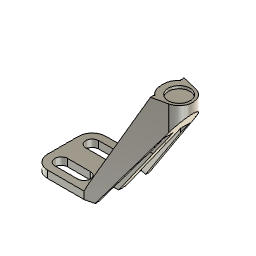
Melta holder for linear init with induction sensor (Autodesk Fusion 360 design; units mm, degrees)
Autodesk Fusion 360 part; units mm, degrees
sketch "Sketch1" plane through (0, 0, 0) normal (0, 0, 1) x (1, 0, 0)
  circle A0 centre (7.5, 6.1469) radius 3.5
  circle A1 centre (7.5, 23.1469) radius 3.5
  circle A2 centre (20, 23.1469) radius 3.5
  circle A3 centre (20, 6.1469) radius 3.5
  line L0 (0, 0) -> (0, 35)
  line L1 (7.5, 26.6469) -> (20, 26.6469)
  line L2 (7.5, 2.6469) -> (20, 2.6469)
  line L3 (7.5, 9.6469) -> (20, 9.6469)
  line L4 (7.5, 19.6469) -> (20, 19.6469)
  circle A4 centre (7.5, 23.1469) radius 7.5
  circle A5 centre (7.5, 6.1469) radius 7.5
  line L5 (0, 23.1469) -> (0, 6)
  circle A6 centre (20, 6.1469) radius 7.5
  circle A7 centre (20, 23.1469) radius 7.5
  line L6 (7.5, 30.6469) -> (20, 30.6469)
  line L7 (7.5, -1.3531) -> (20, -1.3531)
  line L8 (20, -1.3531) -> (27.5, -1.3531)
  line L9 (27.5, -1.3531) -> (27.5, 30.6469)
  line L10 (27.5, 30.6469) -> (20, 30.6469)
  circle A8 centre (63.75, 14.5734) radius 6
  line L11 (13.75, 19.6469) -> (13.75, 2.6469)
  circle A9 centre (63.75, 14.5734) radius 7.5
  line L12 (27.5, -1.3531) -> (65.4115, 7.2598)
  line L13 (27.5, 30.6469) -> (65.4384, 21.8809)
  line L14 (27.5, 14.6469) -> (56.2504, 14.6469)
  line L15 (27.5, 14.6469) -> (27.5, -1.3531)
  arc A10 (56.2504, 14.6469) -> (65.4115, 7.2598) centre (63.75, 14.5734) ccw
  arc A11 (65.4384, 21.8809) -> (56.2504, 14.6469) centre (63.75, 14.5734) ccw
  line L16 (27.5, 14.6469) -> (27.5, 30.6469)
  line L17 (29.5, 16.6469) -> (54.479, 16.6469)
  arc A12 (57.4411, 21.6761) -> (54.479, 16.6469) centre (63.75, 14.5734) ccw
  line L18 (29.5, 28.1321) -> (57.4411, 21.6761)
  line L19 (29.5, 16.6469) -> (29.5, 28.1321)
  line L20 (29.5, 1.1522) -> (57.415, 7.4941)
  arc A13 (54.4474, 12.6469) -> (57.415, 7.4941) centre (63.75, 14.5734) ccw
  line L21 (29.5, 12.6469) -> (54.4474, 12.6469)
  line L22 (29.5, 12.6469) -> (29.5, 1.1522)
  dimension "d1" = 7
  dimension "d2" = 7
  dimension "d3" = 17
  dimension "d4" = 7
  dimension "d5" = 7
  dimension "d8" = 7.5
  dimension "d9" = 7.5
  dimension "d10" = 20
  dimension "d11" = 20
  dimension "d12" = 15
  dimension "d13" = 15
  dimension "d14" = 15
  dimension "d15" = 15
  dimension "d16" = 7.5
  dimension "d17" = 12
  dimension "d19" = 50
  dimension "d20" = 15
  dimension "d21" = 2
  dimension "d22" = 2
  constraint coincident L0.start origin
  constraint vertical L0
  constraint coincident A1 L1.start
  constraint coincident A2 L1.end
  constraint tangent A2 L1
  constraint horizontal L1
  constraint coincident A0 L2.start
  constraint coincident A3 L2.end
  constraint tangent A3 L2
  constraint parallel L1 L2
  constraint coincident A0 L3.start
  constraint coincident A3 L3.end
  constraint tangent A3 L3
  constraint parallel L2 L3
  constraint coincident A1 L4.start
  constraint coincident A2 L4.end
  constraint tangent A2 L4
  constraint parallel L3 L4
  constraint concentric A1 A4
  constraint concentric A0 A5
  constraint coincident A4 L5.start
  constraint coincident L0 L5.end
  constraint tangent A4 L5
  constraint parallel L0 L5
  constraint concentric A3 A6
  constraint concentric A2 A7
  constraint coincident A4 L6.start
  constraint coincident A7 L6.end
  constraint tangent A7 L6
  constraint tangent A4 L6
  constraint coincident A5 L7.start
  constraint coincident A6 L7.end
  constraint tangent A6 L7
  constraint horizontal L7
  constraint parallel L7 L8
  constraint perpendicular L6 L9
  constraint tangent A7 L10
  constraint midpoint L4 L11.start
  constraint midpoint L2 L11.end
  constraint concentric A8 A9
  constraint coincident A9 L12.end
  constraint tangent A9 L12
  constraint coincident A9 L13.end
  constraint tangent A9 L13
  constraint midpoint L9 L14.start
  constraint coincident A9 L14.end
  constraint perpendicular L9 L14
  constraint coincident A8.centre A9.centre
  measures "d1" diameter of A0
  measures "d2" diameter of A1
  measures "d3" vertical distance of A0.centre A1.centre
  measures "d4" diameter of A2
  measures "d5" diameter of A3
  measures "d8" distance of A0.centre L0
  measures "d9" distance of A1.centre L0
  measures "d10" distance of A2.centre L0
  measures "d11" distance of A3.centre L0
  measures "d12" diameter of A4
  measures "d13" diameter of A5
  measures "d14" diameter of A6
  measures "d15" diameter of A7
  measures "d16" distance of L7.end L8.end
  measures "d17" diameter of A8
  measures "d19" distance of A8.centre L11
  measures "d20" diameter of A9
extrude "Extrude1" add sketch "Sketch1" along normal blind 4 contours A0 L2 L3 A5 A6 | L3 A6 L11 | L2 A5 A6 | L3 A5 L11 | A3 L2 L3 A5 A6 | A6 A7 L9 L11 L15 L16 | L0 A4 A5 L5 L11 | A5 A6 L7 | A6 L8 L9 L15 | L4 A4 L11 | A1 L1 L4 A4 A7 | A2 L1 L4 A4 A7 | L4 A7 L11 | A7 L9 L10 L16 | A4 A7 L6 | L1 A4 A7
extrude "Extrude2" add sketch "Sketch1" along normal blind 60 contours L9 A9 L12 L14 L15 A10 | L9 A9 L13 L14 A11 L16 | A9 A10 A11 | A8
chamfer "Chamfer1" distance 27 distance2 56 1 edges at (27.5, 14.6469, 60) measured on face at (61.7658, 13.9292, 60)
chamfer "Chamfer2" distance 57 distance2 2.7 2 edges at (54.5, 5.8064, 60) (54.5, 23.382, 60) measured on face at (28.1667, 15.3135, 5.3827) measured on face at (28.1667, 15.3135, 5.3827)
sketch "Sketch3" plane through (0, -1.3531, 0) normal (0, -1, 0) x (1, 0, 0)
  line L0 (7.5, 0) -> (27.5, 0)
  line L1 (27.5, 0) -> (27.5, 4)
  line L2 (27.5, 4) -> (7.5, 4)
  line L3 (7.5, 4) -> (7.5, 0)
  line L4 (32.4174, -0.0986) -> (71.6605, 55.2443)
  line L5 (71.6605, 55.2443) -> (71.6605, -0.0986)
  line L6 (71.6605, -0.0986) -> (32.4174, -0.0986)
  line L7 (71.6605, 55.2443) -> (78, 55.2443)
  line L8 (78, 55.2443) -> (78, 0)
  line L9 (78, 0) -> (71.6605, 0)
  line L10 (71.6605, 0) -> (71.6605, 55.2443)
  constraint perpendicular L2 L5
  constraint perpendicular L5 L6
  constraint horizontal L7
  constraint vertical L8
  constraint horizontal L9
  constraint vertical L10
extrude "Extrude4" cut sketch "Sketch3" against normal blind 40 contours L4 L5 L6 L10 | L5 L7 L8 L9 L10
sketch "Sketch5" plane through (0, 0, 60) normal (0, 0, 1) x (-1, 0, 0)
  line L0 (-57.2, -23.7845) -> (-57.2, -21.7318)
  line L1 (-57.2, -21.7318) -> (-57.4411, -21.6761)
  arc A0 (-57.4411, -21.6761) -> (-54.5, -16.7385) centre (-63.75, -14.5734) ccw
  line L2 (-54.5, -16.7385) -> (-54.5, -12.4084)
  arc A1 (-54.5, -12.4084) -> (-57.415, -7.4941) centre (-63.75, -14.5734) ccw
  line L3 (-57.415, -7.4941) -> (-57.2, -7.4452)
  line L4 (-57.2, -7.4452) -> (-57.2, -5.3943)
  line L5 (-57.2, -5.3943) -> (-65.4115, -7.2598)
  arc A2 (-65.4115, -7.2598) -> (-65.4384, -21.8809) centre (-63.75, -14.5734) ccw
  line L6 (-65.4384, -21.8809) -> (-57.2, -23.7845)
  circle A3 centre (-63.75, -14.5734) radius 6
  dimension "d36" = 12
  constraint concentric A0 A3
  measures "d36" diameter of A3
extrude "Extrude5" cut sketch "Sketch5" against normal blind 1.5 contours A3
sketch "Sketch6" plane through (0, 0, 0) normal (-1, 0, 0) x (0, -1, 0)
  line L0 (-23.1469, 0) -> (-6.1469, 0)
  line L1 (-6.1469, 0) -> (-6.1469, 4)
  line L2 (-6.1469, 4) -> (-23.1469, 4)
  line L3 (-23.1469, 4) -> (-23.1469, 0)
  line L4 (-16.6486, 29.501) -> (-21.6763, 29.501)
  line L5 (-21.6763, 29.501) -> (-21.6763, 42.1934)
  line L6 (-21.6763, 42.1934) -> (-16.6486, 42.1934)
  line L7 (-16.6486, 42.1934) -> (-16.6486, 29.501)
  line L8 (-12.65, 42.0913) -> (-7.4735, 42.0913)
  line L9 (-7.4735, 42.0913) -> (-7.4735, 26.6395)
  line L10 (-7.4735, 26.6395) -> (-12.65, 26.6395)
  line L11 (-12.65, 26.6395) -> (-12.65, 42.0913)
  dimension "d41" = 15.4518
  constraint horizontal L4
  constraint vertical L5
  constraint horizontal L6
  constraint vertical L7
  constraint horizontal L8
  constraint vertical L9
  constraint horizontal L10
  constraint vertical L11
  measures "d41" distance of L8.end L9.end
extrude "Extrude6" cut sketch "Sketch6" against normal blind 100 contours L4 L5 L6 L7 | L8 L9 L10 L11
equation "d3 = 7 mm + 10 mm"
